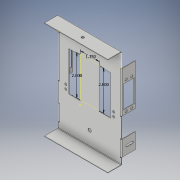
# Autodesk Inventor part: Hew Frame 2017
Saved by Autodesk Inventor 2017 (Build 210142000, 142)
## iProperties
Created: 2016-09-30
Part Number: Hew Frame 2017
Material: Generic
Document SubType Name: Sheet Metal
Designer: Student
Density: 1 g/cm^3
Sheet Metal Rule: Default
Appearance: Default
Flat Pattern Width: 22.5563 cm
Flat Pattern Length: 16.2063 cm
Flat Pattern Area: 365.553 cm^2
Sheet Metal Width: 8.880 in
Sheet Metal Length: 6.380 in
Sheet Metal Area: 56.661 in^2
Author: Student
Autodesk Inventor part; units mm, degrees
note: some values were not read from the file. Chosen so that the rebuilt part matches the saved one: flange form of "Plate5".
ref_plane "YZ Plane" through (0, 0, 0) normal (1, 0, 0) x (0, 1, 0)
ref_plane "XZ Plane" through (0, 0, 0) normal (0, 1, 0) x (-1, 0, 0)
ref_plane "XY Plane" through (0, 0, 0) normal (0, 0, 1) x (1, 0, 0)
sketch "Sketch1" plane through (0, 0, 0) normal (0, 0, 1) x (1, 0, 0)
  line L0 (74.3545, -57.3305) -> (-39.9455, -57.3305)
  line L1 (-39.9455, -57.3305) -> (-39.9455, 120.4695)
  line L2 (-39.9455, 120.4695) -> (74.3545, 120.4695)
  line L3 (74.3545, 120.4695) -> (74.3545, -57.3305)
  line L4 (-39.9455, 57.5322) -> (-39.9455, 77.7975)
  point P0 (0, 0)
  dimension "d0" = 177.8
  dimension "d1" = 114.3
  measures "d0" distance of L0.end L1.end
  measures "d1" distance of L1.end L2.end
extrude "Plate1" add sketch "Sketch1" along normal blind 0.8738
sketch "Sketch2" plane through (-39.9455, 119.5958, 0) normal (0, 1, 0) x (-1, 0, 0)
  line L0 (-114.3, 0) -> (0, 0)
  line L1 (0, 0) -> (0, 25.4)
  line L2 (0, 25.4) -> (-114.3, 25.4)
  line L3 (-114.3, 25.4) -> (-114.3, 0)
  constraints: 6 end point, 1 horizontal, 1 perpendicular, 1 vertical
edge flange "Flange1" height 25.4 angle 90 thickness 0.8738 bend radius 0.8738 thickness toward (0, 1, 0) relief straight relief width 0.8738 relief depth 0.4369 edges at (17.2045, 120.4695, 0.8738) wall of the first edge with corners at (74.3545, 119.5958, 0) (-39.9455, 119.5958, 0) (-39.9455, 119.5958, 25.4) (74.3545, 119.5958, 25.4)
bend "Bend1"
corner "Corner1"
sketch "Sketch3" plane through (73.4807, -57.3305, 0.8738) normal (1, 0, 0) x (0, 1, 0)
  line L0 (150.6525, 0) -> (76.2, 0)
  line L1 (76.2, 0) -> (76.2, -25.4)
  line L2 (76.2, -25.4) -> (150.6525, -25.4)
  line L3 (150.6525, -25.4) -> (150.6525, 0)
  constraints: 8 end point
edge flange "Flange2" height 25.4 angle 90 thickness 0.8738 bend radius 0.8738 thickness toward (1, 0, 0) relief straight relief width 0.8738 relief depth 0.4369 edges at (74.3545, 30.6958, 0) wall of the first edge with corners at (73.4807, 93.322, 0.8738) (73.4807, 18.8695, 0.8738) (73.4807, 18.8695, -24.5262) (73.4807, 93.322, -24.5262)
bend "Bend2"
corner "Corner2"
sketch "Sketch4" plane through (-39.0718, 118.722, 0.8738) normal (-1, 0, 0) x (0, -1, 0)
  line L0 (99.8525, 0) -> (25.4, 0)
  line L1 (25.4, 0) -> (25.4, -25.4)
  line L2 (25.4, -25.4) -> (99.8525, -25.4)
  line L3 (99.8525, -25.4) -> (99.8525, 0)
  constraints: 8 end point
edge flange "Flange3" height 25.4 angle 90 thickness 0.8738 bend radius 0.8738 thickness toward (-1, 0, 0) relief straight relief width 0.8738 relief depth 0.4369 edges at (-39.9455, 30.6958, 0) wall of the first edge with corners at (-39.0718, 18.8695, 0.8738) (-39.0718, 93.322, 0.8738) (-39.0718, 93.322, -24.5262) (-39.0718, 18.8695, -24.5262)
bend "Bend3"
corner "Corner3"
sketch "Sketch5" plane through (74.3545, -56.4567, 0) normal (0, -1, 0) x (1, 0, 0)
  line L0 (-114.3, 0) -> (0, 0)
  line L1 (0, 0) -> (0, 25.4)
  line L2 (0, 25.4) -> (-114.3, 25.4)
  line L3 (-114.3, 25.4) -> (-114.3, 0)
  constraints: 6 end point, 1 horizontal, 1 perpendicular, 1 vertical
edge flange "Flange4" height 25.4 angle 90 thickness 0.8738 bend radius 0.8738 thickness toward (0, -1, 0) relief straight relief width 0.8738 relief depth 0.4369 edges at (17.2045, -57.3305, 0.8738) wall of the first edge with corners at (-39.9455, -56.4567, 0) (74.3545, -56.4567, 0) (74.3545, -56.4567, 25.4) (-39.9455, -56.4567, 25.4)
bend "Bend4"
corner "Corner4"
sketch "Sketch6" plane through (-39.0718, 17.9958, 0.8738) normal (-1, 0, 0) x (0, -1, 0)
  line L0 (35.4787, 0) -> (63.5, 0)
  line L1 (63.5, 0) -> (63.5, -25.4)
  line L2 (63.5, -25.4) -> (35.4787, -25.4)
  line L3 (35.4787, -25.4) -> (35.4787, 0)
  constraints: 8 end point
edge flange "Flange5" height 25.4 angle 90 thickness 0.8738 bend radius 0.8738 thickness toward (-1, 0, 0) relief straight relief width 0.8738 relief depth 0.4369 edges at (-39.9455, -18.7936, 0) wall of the first edge with corners at (-39.0718, -17.4829, 0.8738) (-39.0718, -45.5042, 0.8738) (-39.0718, -45.5042, -24.5262) (-39.0718, -17.4829, -24.5262)
bend "Bend5"
corner "Corner5"
sketch "Sketch7" plane through (73.4807, -55.5829, 0.8738) normal (1, 0, 0) x (0, 1, 0)
  line L0 (10.0787, 0) -> (38.1, 0)
  line L1 (38.1, 0) -> (38.1, -25.4)
  line L2 (38.1, -25.4) -> (10.0787, -25.4)
  line L3 (10.0787, -25.4) -> (10.0787, 0)
  constraints: 8 end point
edge flange "Flange6" height 25.4 angle 90 thickness 0.8738 bend radius 0.8738 thickness toward (1, 0, 0) relief straight relief width 0.8738 relief depth 0.4369 edges at (74.3545, -18.7936, 0) wall of the first edge with corners at (73.4807, -45.5042, 0.8738) (73.4807, -17.4829, 0.8738) (73.4807, -17.4829, -24.5262) (73.4807, -45.5042, -24.5262)
bend "Bend6"
corner "Corner6"
sketch "Sketch8" plane through (0, 0, 0.8738) normal (0, 0, 1) x (1, 0, 0)
  point P0 (0, 0)
sketch "Sketch9" plane through (-39.9455, 119.5958, 25.4) normal (0, -1, 0) x (1, 0, 0)
  line L0 (0, 0) -> (0, -23.6525) projected
  line L1 (114.3, 0) -> (0, 0) projected
  circle A0 centre (57.15, -11.8262) radius 2.3495
  point P0 (39.9455, -25.4)
  dimension "d72" = 4.699
  constraints: 1 centre point
  measures "d72" diameter of A0
extrude "Extrusion1" cut sketch "Sketch9" against normal blind 25.4
sketch "Sketch10" plane through (0, 0, 0.8738) normal (0, 0, 1) x (1, 0, 0)
  line L0 (-39.9455, 94.1958) -> (-39.9455, 118.722) projected
  line L1 (74.3545, 118.722) -> (74.3545, 94.1958) projected
  line L2 (72.1701, 93.322) -> (72.1701, 94.1958) projected
  line L3 (-37.7611, 94.1958) -> (-37.7611, 93.322) construction
  line L4 (0.0595, 78.8847) -> (0.0595, 7.7647) construction
  line L5 (34.3495, 78.8847) -> (34.3495, 7.7647) construction
  line L6 (0.0595, 78.8847) -> (34.3495, 78.8847) construction
  line L7 (0.0595, 7.7647) -> (0.0595, 78.8847) construction
  line L8 (0.0595, 7.7647) -> (34.3495, 7.7647) construction
  point P0 (0, 0)
  dimension "d135" = 71.12
  dimension "d136" = 71.12
  dimension "d137" = 34.29
  constraints: 10 end point, 2 horizontal, 2 vertical
  measures "d135" distance of L4.start L4.end
  measures "d136" distance of L5.start L5.end
  measures "d137" distance of L4.start L5.start
sketch "Sketch11" plane through (0, 0, 0.8738) normal (0, 0, 1) x (1, 0, 0)
  line L0 (0, 77.6598) -> (-20.32, 77.6598)
  line L1 (-20.32, 77.6598) -> (-20.32, 6.5398)
  line L2 (-20.32, 6.5398) -> (0, 6.5398)
  line L3 (0, 6.5398) -> (0, 77.6598)
  line L4 (34.3338, 77.6598) -> (54.6538, 77.6598)
  line L5 (54.6538, 77.6598) -> (54.6538, 6.5398)
  line L6 (54.6538, 6.5398) -> (34.3338, 6.5398)
  line L7 (34.3338, 6.5398) -> (34.3338, 77.6598)
  point P0 (0, 0)
  dimension "d78" = 71.12
  dimension "d79" = 71.12
  dimension "d80" = 20.32
  dimension "d81" = 20.32
  constraints: 16 end point, 4 parallel, 2 horizontal, 2 perpendicular
  measures "d78" distance of L6.end L4.start
  measures "d79" distance of L2.end L0.start
  measures "d80" distance of L0.start L0.end
  measures "d81" distance of L4.start L4.end
extrude "Cut1" cut sketch "Sketch11" against normal blind 0.8738
sketch "Sketch20" plane through (74.3545, 18.8695, -24.5262) normal (1, 0, 0) x (0, 0, -1)
  line L0 (-21.7983, 8.5475) -> (-1.8847, 8.5475)
  line L1 (-1.8847, 8.5475) -> (-1.8847, 49.0475)
  line L2 (-1.8847, 49.0475) -> (-21.7983, 49.0475)
  line L3 (-21.7983, 49.0475) -> (-21.7983, 8.5475)
  line L4 (-23.6525, 74.4525) -> (-23.6525, 0) projected
  point P0 (-24.5262, -18.8695)
  dimension "d139" = 19.9136
  dimension "d140" = 40.5
  dimension "d141" = 1.8542
  constraints: 8 end point, 2 parallel, 1 horizontal, 1 perpendicular
  measures "d139" distance of L0.start L0.end
  measures "d140" distance of L2.end L0.start
  measures "d141" distance between parallel lines of L3 L4
extrude "Extrusion2" cut sketch "Sketch20" against normal blind 127
sketch "Sketch21" plane through (74.3545, -45.5042, -24.5262) normal (1, 0, 0) x (0, 0, -1)
  line L0 (-5.8174, 14.0106) -> (-15.2947, 14.0106) construction
  line L1 (-5.8174, 11.9294) -> (-15.2947, 11.9294)
  line L2 (-15.2947, 16.0919) -> (-5.8174, 16.0919)
  arc A0 (-5.8174, 11.9294) -> (-5.8174, 16.0919) centre (-5.8174, 14.0106) ccw
  arc A1 (-15.2947, 16.0919) -> (-15.2947, 11.9294) centre (-15.2947, 14.0106) ccw
  point P0 (-24.5262, 45.5042)
  point P1 (-10.556, 14.0106)
  dimension "d144" = 13.6398
  constraints: 8 end point, 4 point on circle, 4 tangent, 2 centre point, 1 horizontal, 1 midpoint, 1 parallel
extrude "Extrusion3" cut sketch "Sketch21" against normal blind 127
sketch "Sketch22" plane through (74.3545, 18.8695, -24.5262) normal (1, 0, 0) x (0, 0, -1)
  line L0 (-21.7983, 8.5475) -> (-21.7983, 49.0475) projected
  line L1 (-21.7983, 8.5475) -> (-1.8703, 8.5475) construction
  line L2 (-1.8703, 8.5475) -> (-1.8703, 1.1305) construction
  line L3 (-1.8703, 1.1305) -> (-21.7983, 1.1305) construction
  line L4 (-21.7983, 1.1305) -> (-21.7983, 8.5475) construction
  line L5 (-21.7983, 49.0475) -> (-1.8847, 49.0475) construction
  line L6 (-21.7983, 49.0475) -> (-1.8703, 49.0475) construction
  line L7 (-1.8703, 49.0475) -> (-1.8703, 56.4645) construction
  line L8 (-1.8703, 56.4645) -> (-21.7983, 56.4645) construction
  line L9 (-21.7983, 56.4645) -> (-21.7983, 49.0475) construction
  line L10 (-1.8847, 8.5475) -> (-21.7983, 8.5475) construction
  line L11 (-11.8415, 8.5475) -> (-11.8343, 1.1305) construction
  circle A0 centre (-16.8408, 3.9755) radius 2.159
  circle A1 centre (-6.8305, 3.9755) radius 2.159
  line L12 (-11.8343, 49.0475) -> (-11.8343, 56.4645) construction
  circle A2 centre (-16.8417, 53.6195) radius 2.159
  circle A3 centre (-6.8305, 53.6195) radius 2.159
  point P0 (-24.5262, -18.8695)
  dimension "d147" = 7.417
  dimension "d149" = 4.318
  dimension "d150" = 5.0038
  dimension "d151" = 4.318
  dimension "d152" = 5.0038
  dimension "d178" = 4.572
  dimension "d179" = 4.572
  dimension "d180" = 4.572
  dimension "d181" = 4.572
  constraints: 20 end point, 4 centre point, 4 midpoint, 4 parallel, 2 horizontal, 2 perpendicular
  measures "d147" distance of L3.end L0.start
  measures "d149" diameter of A0
  measures "d150" distance from line of L11 A0.centre
  measures "d151" diameter of A1
  measures "d152" horizontal distance of L11.end A1.centre
  measures "d178" distance from line of L5 A3.centre
  measures "d179" distance from line of L5 A2.centre
  measures "d180" distance from line of A1.centre L1
  measures "d181" distance from line of L10 A0.centre
extrude "Extrusion4" cut sketch "Sketch22" against normal blind 127
sketch "Sketch23" plane through (0, 0, 0.8738) normal (0, 0, 1) x (1, 0, 0)
  line L0 (-36.9229, 24.3198) -> (71.3319, 24.3198)
  line L1 (-20.32, 6.5398) -> (-20.32, 77.6598) projected
  line L2 (-39.9455, -16.6092) -> (-39.9455, 17.9958) projected
  line L3 (0, 6.5398) -> (-20.32, 6.5398) projected
  line L4 (-36.9229, 6.5398) -> (-20.32, 6.5398)
  circle A0 centre (-25.9755, 11.6198) radius 1.9939
  line L5 (-36.9229, 24.3198) -> (-36.9229, 6.5398)
  circle A1 centre (-25.9755, 19.2398) radius 1.9939
  circle A2 centre (60.3845, 19.2398) radius 1.9939
  circle A3 centre (60.3845, 11.6198) radius 1.9939
  point P0 (0, 0)
  dimension "d162" = 108.2548
  dimension "d163" = 3.0226
  dimension "d164" = 16.6029
  dimension "d165" = 17.78
  dimension "d166" = 3.9878
  dimension "d167" = 3.9878
  dimension "d168" = 10.9474
  dimension "d169" = 10.9474
  dimension "d170" = 7.62
  dimension "d171" = 5.08
  dimension "d172" = 3.9878
  dimension "d173" = 3.9878
  dimension "d174" = 10.9474
  dimension "d175" = 10.9474
  constraints: 6 end point, 4 centre point, 1 collinear, 1 horizontal
  measures "d162" distance of L0.start L0.end
  measures "d163" distance from line of L0.start L2
  measures "d164" distance of L4.start L1.start
  measures "d165" distance of L0.start L4.start
  measures "d166" diameter of A0
  measures "d167" diameter of A1
  measures "d168" distance from line of L5 A1.centre
  measures "d169" horizontal distance of L4.start A0.centre
  measures "d170" distance of A0.centre A1.centre
  measures "d171" distance from line of L0 A1.centre
  measures "d172" diameter of A2
  measures "d173" diameter of A3
  measures "d174" horizontal distance of L0.end A2.centre
  measures "d175" horizontal distance of L0.end A3.centre
extrude "Extrusion5" cut sketch "Sketch23" against normal blind 25.4 contours A0 | A1 | A2 | A3
sketch "Sketch25" plane through (0, 0, 0.8738) normal (0, 0, 1) x (1, 0, 0)
  circle A0 centre (17.2045, -31.0567) radius 2.9972
  line L0 (-39.9455, -55.5829) -> (-39.9455, -46.378) projected
  line L1 (-39.9455, -56.4567) -> (74.3545, -56.4567) projected
  point P0 (0, 0)
  dimension "d183" = 5.9944
  constraints: 1 centre point
  measures "d183" diameter of A0
extrude "Extrusion6" cut sketch "Sketch25" against normal through all
equation "\"d82\" = Thickness"
equation "\"d4\" = BendReliefWidth"
equation "\"d5\" = BendReliefDepth"
equation "\"d6\" = MinimumRemnant"
equation "\"d7\" = BendRadius"
equation "\"d10\" = Thickness"
equation "\"d11\" = CornerReliefSize"
equation "\"d12\" = GapSize"
equation "\"d13\" = JacobiRadiusSize"
equation "\"d14\" = BendReliefWidth"
equation "\"d15\" = BendReliefDepth"
equation "\"d16\" = MinimumRemnant"
equation "\"d17\" = BendRadius"
equation "\"d22\" = JacobiRadiusSize"
equation "\"d23\" = CornerReliefSize"
equation "\"d24\" = GapSize"
equation "\"d25\" = JacobiRadiusSize"
equation "\"d26\" = BendReliefWidth"
equation "\"d27\" = BendReliefDepth"
equation "\"d28\" = MinimumRemnant"
equation "\"d29\" = BendRadius"
equation "\"d34\" = JacobiRadiusSize"
equation "\"d35\" = CornerReliefSize"
equation "\"d36\" = GapSize"
equation "\"d37\" = JacobiRadiusSize"
equation "\"d38\" = BendReliefWidth"
equation "\"d39\" = BendReliefDepth"
equation "\"d40\" = MinimumRemnant"
equation "\"d41\" = BendRadius"
equation "\"d44\" = JacobiRadiusSize"
equation "\"d45\" = CornerReliefSize"
equation "\"d46\" = GapSize"
equation "\"d47\" = JacobiRadiusSize"
equation "\"d48\" = BendReliefWidth"
equation "\"d49\" = BendReliefDepth"
equation "\"d50\" = MinimumRemnant"
equation "\"d51\" = BendRadius"
equation "\"d56\" = JacobiRadiusSize"
equation "\"d57\" = CornerReliefSize"
equation "\"d58\" = GapSize"
equation "\"d59\" = JacobiRadiusSize"
equation "\"d60\" = BendReliefWidth"
equation "\"d61\" = BendReliefDepth"
equation "\"d62\" = MinimumRemnant"
equation "\"d63\" = BendRadius"
equation "\"d68\" = JacobiRadiusSize"
equation "\"d69\" = CornerReliefSize"
equation "\"d70\" = GapSize"
equation "\"d71\" = JacobiRadiusSize"
equation "\"BendRadius\" = Thickness"
equation "\"BendReliefWidth\" = Thickness"
equation "\"BendReliefDepth\" = 0.5 * Thickness"
equation "\"CornerReliefSize\" = 4 * Thickness"
equation "\"MinimumRemnant\" = 2 * Thickness"
equation "\"TransitionRadius\" = BendRadius"
equation "\"JacobiRadiusSize\" = Thickness"
equation "\"GapSize\" = Thickness"
equation "\"d3\" = BendRadius"
equation "\"Thickness\" = 0.87376"
body "Solid1"
